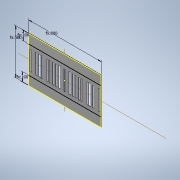
# Autodesk Inventor part: ferrite_layer_dex_1R1
Saved by Autodesk Inventor 2021 (Build 250183000, 183)
## iProperties
Created: 2021-01-27
Part Number: ferrite_layer_dex_1R1
Material: Generic
Document SubType Name: Modeling
Designer: pduy110
Density: 1 g/cm^3
Appearance: Smooth - Medium Gray
Author: pduy110
Autodesk Inventor part; units mm, degrees
ref_plane "YZ Plane" through (0, 0, 0) normal (1, 0, 0) x (0, 1, 0)
ref_plane "XZ Plane" through (0, 0, 0) normal (0, 1, 0) x (-1, 0, 0)
ref_plane "XY Plane" through (0, 0, 0) normal (0, 0, 1) x (1, 0, 0)
sketch "ferrite_layer_outline_sketch" plane through (0, 0, 0) normal (0, 0, 1) x (1, 0, 0)
  line L0 (-400, 250) -> (400, 250)
  line L1 (400, 250) -> (400, -250)
  line L2 (400, -250) -> (-400, -250)
  line L3 (-400, -250) -> (-400, 250)
  line L4 (0, 250) -> (0, -250) construction
  line L5 (0, 136.1953) -> (0, -273.5408) construction
  line L6 (0, 250) -> (0, -250)
  point P0 (0, 0)
  point P1 (0, 0)
  point P2 (0, 0)
  dimension "d85" = 800
  dimension "d86" = 500
  constraints: 14 end point, 4 midpoint, 2 parallel, 2 point on line, 1 coincident, 1 collinear, 1 horizontal, 1 perpendicular
  measures "d85" distance between parallel lines of L1 L3
  measures "d86" distance between parallel lines of L2 L0
extrude "Sheet Extrude" add sketch "ferrite_layer_outline_sketch" along normal blind 4
ref_plane "acrylic_sheet_plane" through (0, 0, 4) normal (0, 0, 1) x (1, 0, 0)
sketch "Sketch4" plane through (0, 0, 4) normal (0, 0, 1) x (1, 0, 0)
  line L0 (-385.5, 109) -> (-370.5, 109)
  line L1 (-370.5, 109) -> (-370.5, -109)
  line L2 (-370.5, -109) -> (-385.5, -109)
  line L3 (-385.5, -109) -> (-385.5, 109)
  line L4 (-12.6534, 0) -> (47.471, 0)
  line L5 (-400, 250) -> (-400, -250) projected
  line L6 (400, 250) -> (-400, 250) projected
  line L7 (-400, -250) -> (400, -250) projected
  point P0 (0, 0)
  point P1 (-385.5, 0)
  point P2 (-400, 0)
  dimension "d43" = 15
  dimension "d44" = 218
  dimension "d45" = 14.5
  constraints: 10 end point, 2 horizontal, 2 parallel, 2 point on line, 1 midpoint, 1 perpendicular, 2 other
  measures "d43" distance between parallel lines of L1 L3
  measures "d44" distance between parallel lines of L2 L0
extrude "Extrusion9" cut sketch "Sketch4" against normal through all
pattern_linear "Rectangular Pattern 7 fer" count 7 spacing 126 along (1, 0, 0) of "Extrusion9"
pattern_linear "Rectangular Pattern 8 fer" count 8 spacing 108 along (1, 0, 0) of "Extrusion9"
pattern_linear "pattern_test_#_of_ferrites 9 fer" count 9 spacing 94.5 along (1, 0, 0) of "Extrusion9"
pattern_linear "Rectangular Pattern 10 fer" [suppressed]
pattern_linear "Rectangular Pattern 13" count 13 spacing 63 along (1, 0, 0) of "Extrusion9"
sketch "Sketch5" plane through (0, 0, 4) normal (0, 0, 1) x (1, 0, 0)
  line L0 (-400, 250) -> (-400, -250) projected
  line L1 (-400, 150) -> (400, 150)
  line L2 (400, -250) -> (400, 250) projected
  line L3 (400, 250) -> (-400, 250) projected
  line L4 (-400, -250) -> (400, -250) projected
  line L5 (-400, -150) -> (400, -150)
  point P0 (0, 0)
  dimension "d66" = 100
  dimension "d68" = 100
  constraints: 4 end point, 2 point on line, 1 horizontal, 1 perpendicular, 3 other
  measures "d66" distance between parallel lines of L3 L1
  measures "d68" distance between parallel lines of L4 L5
equation "\"d85\" = track_length"
equation "\"d86\" = track_width"
equation "\"d43\" = ferrite_width"
equation "\"d44\" = ferrite_length"
equation "\"d45\" = gap_distance"
equation "\"d50\" = parameter_5"
equation "\"d62\" = test_parameter_5"
equation "\"track_length\" = 800"
equation "\"track_width\" = 500"
equation "\"gap_distance\" = 14.5"
equation "\"ferrite_length\" = 218"
equation "\"ferrite_width\" = 15"
equation "\"ferrite_height\" = 8"
equation "\"acrylic_sheet_8mm\" = 8"
equation "\"parameter_5\" = 126"
equation "\"test_parameter_5\" = 94.5"
body "Solid8"
